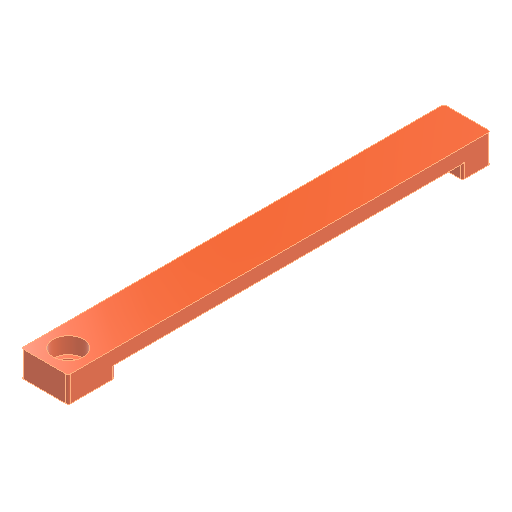
# Autodesk Inventor part: VEJ-00-015
Saved by Autodesk Inventor 2026.1 (Build 301233000, 233)
## iProperties
Company: Venttos
Created: 2025-08-20
Part Number: VEJ-00-015
Checked By: Antonio Lucas
Engr Approved By: Antonio Lucas
Material: Fenolite OR
Document SubType Name: Modeling
Mfg Approved By: Anderson Oliveira
Designer: Willian Pinheiro
Mass: 4.11271 g
Surface Area: 26.5621 cm^2
Volume: 2.98023 cm^3
Density: 1.38 g/cm^3
Appearance: Suave - Laranja claro
Project: VEJ-00
Description: Clamp Central Palete
Dimensões: 6 x 10 x 90 mm
Total: 1
Author: Willian Pinheiro
Title: Palete
Revision Number: 00
Autodesk Inventor part; units mm, degrees
ref_plane "YZ Plane" through (0, 0, 0) normal (1, 0, 0) x (0, 1, 0)
ref_plane "XZ Plane" through (0, 0, 0) normal (0, 1, 0) x (-1, 0, 0)
ref_plane "XY Plane" through (0, 0, 0) normal (0, 0, 1) x (1, 0, 0)
sketch "Esboço1" plane through (0, 0, 0) normal (0, 0, 1) x (1, 0, 0)
  line L0 (-119, 0) -> (119, 0) construction
  line L1 (0, -159) -> (0, 79) construction
  line L2 (-5, 45) -> (5, 45)
  line L3 (5, 45) -> (5, -45)
  line L4 (5, -45) -> (-5, -45)
  line L5 (-5, -45) -> (-5, 45)
  circle A0 centre (0, -40) radius 5
  circle A1 centre (0, 40) radius 5
  circle A2 centre (0, 42) radius 3
  line L6 (-5, 39) -> (5, 39)
  line L7 (5, 39) -> (5, -35)
  line L8 (5, -35) -> (-5, -35)
  line L9 (-5, -35) -> (-5, 39)
  circle A3 centre (0, -40) radius 85
  point P0 (0, 0)
  point P1 (5, 39)
  point P2 (-5, -35)
  dimension "d0" = 10
  dimension "d2" = 85
  dimension "d3" = 90
  dimension "d4" = 6
  dimension "d20" = 170
  constraints: 16 end point, 9 tangent, 4 centre point, 4 parallel, 3 point on line, 2 horizontal, 2 perpendicular, 1 coincident, 1 midpoint, 2 other
  measures "d0" distance between parallel lines of L3 L5
  measures "d2" distance from line of A0.centre L2
  measures "d3" distance between parallel lines of L2 L4
  measures "d4" diameter of A2
  measures "d20" diameter of A3
extrude "Extrusão1" add sketch "Esboço1" against normal blind 6 contours L2 A3 L5 | A3 L3 A1 | A2 L6 A1 | A1 L6 A2 | A2 | L2 L3 A3 | A1 L5 A3 | L3 L6 A1 | A1 L6 L5 | L6 A1 | L3 L8 L5 L6 A1 | L3 A0 L8 | L8 A0 L5 | A0 | L3 L4 A0 | A0 L4 L5
extrude "Extrusão2" cut sketch "Esboço1" along normal blind 0.5 from surface at -6 contours L6 A1 | L3 L8 L5 L6 A1 | L3 A0 L8 | L8 A0 L5 | A0 | L3 L4 A0 | A0 L4 L5
extrude "Extrusão3" cut sketch "Esboço1" along normal blind 2.5 from surface at -5.5 contours L6 A1 | L3 L8 L5 L6 A1
hole "Furo1" at (0, -40, 0) direction (0, 0, -1) diameter 4.5 end through all counterbore diameter 6.5 counterbore depth 3.5 clearance for "Socket Head Cap Screw ISO 4762" size "M4" standard "ISO"
fillet "Arredondamento1" radius 0.5 8 edges at (-5, 39, -4.5) (5, 39, -4.5) (-5, 45, -3) (5, 45, -3) (-5, -35, -4.25) (-5, -45, -2.75) (5, -45, -2.75) (5, -35, -4.25)
